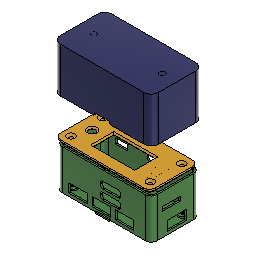
Raspi Zero 2W Case Zero4U V1.0 (Autodesk Fusion 360 design; units mm, degrees)
Autodesk Fusion 360 part; units mm, degrees
sketch "Skizze1" plane through (0, 0, 0) normal (0, 0, 1) x (1, 0, 0)
  line L0 (3, 0) -> (64, 0)
  line L1 (67, 3) -> (67, 30)
  line L2 (64, 33) -> (3, 33)
  line L3 (0, 30) -> (0, 3)
  arc A0 (3, 33) -> (0, 30) centre (3, 30) ccw
  arc A1 (67, 30) -> (64, 33) centre (64, 30) ccw
  arc A2 (64, 0) -> (67, 3) centre (64, 3) ccw
  arc A3 (0, 3) -> (3, 0) centre (3, 3) ccw
  line L4 (-1.2, 30) -> (-1.2, 3)
  arc A4 (-1.2, 3) -> (3, -1.2) centre (3, 3) ccw
  line L5 (3, -1.2) -> (64, -1.2)
  arc A5 (64, -1.2) -> (68.2, 3) centre (64, 3) ccw
  line L6 (68.2, 3) -> (68.2, 30)
  arc A6 (68.2, 30) -> (64, 34.2) centre (64, 30) ccw
  line L7 (64, 34.2) -> (3, 34.2)
  arc A7 (3, 34.2) -> (-1.2, 30) centre (3, 30) ccw
  point P0 (67, 0)
  point P1 (0, 33)
  dimension "d7" = 67
  dimension "d8" = 33
  dimension "d9" = 3
  dimension "d10" = 1.2
  constraint horizontal L0
  constraint vertical L1
  constraint horizontal L2
  constraint vertical L3
  constraint coincident P1 L2
  constraint coincident P1 L3
  constraint tangent L2 A0
  constraint tangent L3 A0
  constraint tangent L1 A1
  constraint tangent L2 A1
  constraint equal A0 A1
  constraint coincident P0 L0
  constraint coincident P0 L1
  constraint tangent L0 A2
  constraint tangent L1 A2
  constraint equal A0 A2
  constraint coincident origin L0
  constraint coincident origin L3
  constraint tangent L0 A3
  constraint tangent L3 A3
  constraint equal A0 A3
  measures "d7" distance of origin P0
  measures "d8" distance of origin P1
  measures "d9" radius of A0
extrude "Extrusion2" add sketch "Skizze1" against normal blind 1.2 contours L0 L1 L2 L3 A0 A1 A2 A3 | L4 A4 L5 A5 L6 A6 L7 A7 makes body 1
extrude "Extrusion3" add sketch "Skizze1" along normal blind 28 bodies 1
ref_plane "Arbeitsebene1" through (70.2, 0, 0) normal (1, 0, 0) x (0, 1, 0)
sketch "Skizze2" plane through (70.2, 0, 0) normal (1, 0, 0) x (0, 1, 0)
  line L0 (7, 18.5) -> (20, 18.5)
  line L1 (20, 18.5) -> (20, 15.5)
  line L2 (20, 15.5) -> (7, 15.5)
  line L3 (7, 15.5) -> (7, 18.5)
  line L4 (3, 0) -> (30, 0)
  line L5 (10.75, 8) -> (24.25, 8)
  line L6 (24.25, 8) -> (24.25, 1)
  line L7 (24.25, 1) -> (10.75, 1)
  line L8 (10.75, 1) -> (10.75, 8)
  line L9 (17.5, 35) -> (17.5, -5) construction
  point P0 (33, 0)
  dimension "d18" = 15.5
  dimension "d19" = 7
  dimension "d20" = 13.5
  dimension "d23" = 17.5
  dimension "d27" = 7
  dimension "d60" = 3
  dimension "d140" = 1
  constraint horizontal L0
  constraint vertical L1
  constraint horizontal L2
  constraint vertical L3
  constraint horizontal L5
  constraint vertical L6
  constraint horizontal L7
  constraint vertical L8
  constraint perpendicular L7 L9
  measures "d18" distance of L2.end L4
  measures "d19" horizontal distance of origin L2.end
  measures "d20" distance of L5.start L5.end
  measures "d23" distance of origin L9
  measures "d27" distance of L5.end L6.end
  measures "d60" distance of L0 L2
  measures "d140" distance of L4 L7
extrude "Extrusion4" cut sketch "Skizze2" against normal blind 3.2 bodies 1
ref_plane "Arbeitsebene2" through (-3.2, 0, 0) normal (1, 0, 0) x (0, 1, 0)
sketch "Skizze3" plane through (-3.2, 0, 0) normal (1, 0, 0) x (0, 1, 0)
  line L0 (16, 30) -> (16, -12) construction
  line L1 (23, 17) -> (25, 17)
  line L2 (25, 17) -> (25, 22)
  line L3 (25, 22) -> (23, 22)
  line L4 (23, 22) -> (23, 17)
  point P0 (33, 0)
  dimension "d166" = 17
  constraint horizontal L1
  constraint vertical L2
  constraint horizontal L3
  constraint vertical L4
  measures "d166" vertical distance of origin L1.end
extrude "Extrusion5" cut sketch "Skizze3" along normal blind 3.2 bodies 1
ref_plane "Arbeitsebene3" through (33.5, 36.2, 13.4) normal (0, 1, 0) x (1, 0, 0)
sketch "Skizze4" plane through (0, 36.2, 0) normal (0, 1, 0) x (1, 0, 0)
  line L0 (33.5, -32) -> (33.5, 14) construction
  line L1 (44, -21) -> (33, -21)
  line L2 (31, -19) -> (31, -18)
  line L3 (33, -16) -> (44, -16)
  line L4 (46, -18) -> (46, -19)
  line L5 (67, 0) -> (67, -28)
  line L6 (64, 0) -> (3, 0)
  line L7 (44, -9) -> (33, -9)
  line L8 (31, -11) -> (31, -12)
  line L9 (33, -14) -> (44, -14)
  line L10 (46, -12) -> (46, -11)
  arc A0 (44, -21) -> (46, -19) centre (44, -19) ccw
  arc A1 (31, -19) -> (33, -21) centre (33, -19) ccw
  arc A2 (33, -16) -> (31, -18) centre (33, -18) ccw
  arc A3 (46, -18) -> (44, -16) centre (44, -18) ccw
  arc A4 (46, -11) -> (44, -9) centre (44, -11) ccw
  arc A5 (33, -9) -> (31, -11) centre (33, -11) ccw
  arc A6 (31, -12) -> (33, -14) centre (33, -12) ccw
  arc A7 (44, -14) -> (46, -12) centre (44, -12) ccw
  line L11 (17, -19) -> (8, -19)
  line L12 (8, -19) -> (8, -15)
  line L13 (8, -15) -> (17, -15)
  line L14 (17, -15) -> (17, -19)
  line L15 (0, 0) -> (0, -28)
  point P0 (46, -21)
  point P1 (31, -21)
  point P2 (46, -16)
  point P3 (46, -9)
  point P4 (31, -9)
  dimension "d33" = 33.5
  dimension "d61" = 15
  dimension "d62" = 5
  dimension "d63" = 21
  dimension "d64" = 16
  dimension "d65" = 15
  dimension "d66" = 21
  dimension "d69" = 2
  dimension "d154" = 9
  dimension "d155" = 9
  dimension "d156" = 4
  dimension "d157" = 15
  dimension "d158" = 8
  constraint horizontal L1
  constraint vertical L2
  constraint horizontal L3
  constraint vertical L4
  constraint horizontal L7
  constraint vertical L8
  constraint horizontal L9
  constraint vertical L10
  constraint coincident P0 L1
  constraint coincident P0 L4
  constraint tangent L1 A0
  constraint tangent L4 A0
  constraint coincident P1 L1
  constraint coincident P1 L2
  constraint tangent L1 A1
  constraint tangent L2 A1
  constraint equal A0 A1
  constraint tangent L2 A2
  constraint tangent L3 A2
  constraint equal A0 A2
  constraint coincident P2 L3
  constraint coincident P2 L4
  constraint tangent L3 A3
  constraint tangent L4 A3
  constraint equal A0 A3
  constraint coincident P3 L7
  constraint coincident P3 L10
  constraint tangent L7 A4
  constraint tangent L10 A4
  constraint equal A0 A4
  constraint coincident P4 L7
  constraint coincident P4 L8
  constraint tangent L7 A5
  constraint tangent L8 A5
  constraint equal A0 A5
  constraint tangent L8 A6
  constraint tangent L9 A6
  constraint equal A0 A6
  constraint tangent L9 A7
  constraint tangent L10 A7
  constraint equal A0 A7
  constraint horizontal L11
  constraint vertical L12
  constraint horizontal L13
  constraint vertical L14
  measures "d33" distance of L15.start L0
  measures "d61" distance of P0 P1
  measures "d62" distance of P0 P2
  measures "d63" distance of L4 L5
  measures "d64" distance of L3 L6
  measures "d65" distance of P3 P4
  measures "d66" distance of L5 L10
  measures "d69" radius of A0
  measures "d154" distance of L6 L7.start
  measures "d155" distance of L11.start L11.end
  measures "d156" distance of L11.start L13.end
  measures "d157" distance of L6 L12.end
  measures "d158" distance of L11.end L15
extrude "Extrusion7" cut sketch "Skizze4" against normal blind 3.2 contours L1 L2 L3 L4 A0 A1 A2 A3 | L7 L8 L9 L10 A4 A5 A6 A7 bodies 1
sketch "Skizze5" plane through (0, 0, 0) normal (0, 0, 1) x (1, 0, 0)
  line L0 (1, 31.5) -> (66, 31.5)
  line L1 (66, 31.5) -> (66, 1.5)
  line L2 (66, 1.5) -> (1, 1.5)
  line L3 (1, 1.5) -> (1, 31.5)
  circle A0 centre (4.5, 28) radius 2.5
  circle A1 centre (62.5, 28) radius 2.5
  circle A2 centre (4.5, 5) radius 2.5
  circle A3 centre (62.5, 5) radius 2.5
  circle A4 centre (4.5, 28) radius 3.5
  circle A5 centre (62.5, 28) radius 3.5
  circle A6 centre (4.5, 5) radius 3.5
  circle A7 centre (62.5, 5) radius 3.5
  circle A8 centre (4.5, 28) radius 1.35
  circle A9 centre (62.5, 28) radius 1.35
  circle A10 centre (62.5, 5) radius 1.35
  circle A11 centre (4.5, 5) radius 1.35
  dimension "d40" = 30
  dimension "d41" = 65
  dimension "d42" = 5
  dimension "d43" = 3.5
  dimension "d44" = 3.5
  dimension "d45" = 5
  dimension "d46" = 3.5
  dimension "d47" = 3.5
  dimension "d48" = 5
  dimension "d49" = 3.5
  dimension "d50" = 3.5
  dimension "d51" = 5
  dimension "d52" = 3.5
  dimension "d53" = 3.5
  dimension "d54" = 7
  dimension "d55" = 7
  dimension "d56" = 7
  dimension "d57" = 7
  dimension "d114" = 2.7
  dimension "d115" = 2.7
  dimension "d116" = 2.7
  dimension "d117" = 2.7
  dimension "d162" = 1.5
  dimension "d165" = 1
  constraint horizontal L0
  constraint vertical L1
  constraint horizontal L2
  constraint vertical L3
  constraint concentric A0 A4
  constraint concentric A1 A5
  constraint concentric A2 A6
  constraint concentric A3 A7
  constraint concentric A4 A8
  constraint concentric A1 A9
  constraint concentric A7 A10
  constraint concentric A6 A11
  measures "d40" distance of L0.start L2.end
  measures "d41" distance of L1.end L2.end
  measures "d42" diameter of A0
  measures "d43" distance of L3 A0.centre
  measures "d44" distance of L0 A0.centre
  measures "d45" diameter of A1
  measures "d46" distance of L0 A1.centre
  measures "d47" distance of L1 A1.centre
  measures "d48" diameter of A2
  measures "d49" distance of L3 A2.centre
  measures "d50" distance of L2 A2.centre
  measures "d51" diameter of A3
  measures "d52" distance of L2 A3.centre
  measures "d53" distance of L1 A3.centre
  measures "d54" diameter of A4
  measures "d55" diameter of A5
  measures "d56" diameter of A6
  measures "d57" diameter of A7
  measures "d114" diameter of A8
  measures "d115" diameter of A11
  measures "d116" diameter of A10
  measures "d117" diameter of A9
  measures "d162" vertical distance of origin L2.end
  measures "d165" horizontal distance of origin L2.end
extrude "Extrusion18" add sketch "Skizze5" along normal blind 1 contours A4 | A5 | A6 | A7 | A0 | A1 | A2 | A3 bodies 1
extrude "Extrusion19" cut sketch "Skizze5" against normal blind 1.2 contours A8 | A9 | A10 | A11 bodies 1
chamfer "Fase4" distance 1.4 angle 45 2 edges at (61.2414, 4.5118, -1.2) (3.2414, 27.5118, -1.2) on bodies 1
chamfer "Fase4" distance 1.4 angle 45 2 edges at (61.2414, 27.5118, -1.2) (3.2414, 4.5118, -1.2) on bodies 1
extrude "Extrusion9" cut sketch "Skizze4" against normal blind 42 contours L1 L2 L3 L4 A0 A1 A2 A3 | L7 L8 L9 L10 A4 A5 A6 A7 bodies 1
ref_plane "Arbeitsebene4" through (33.5, 16.5, 30) normal (0, 0, 1) x (1, 0, 0)
sketch "Skizze6" plane through (0, 0, 30) normal (0, 0, 1) x (1, 0, 0)
  arc A0 (3, 34.2) -> (-1.2, 30) centre (3, 30) ccw
  line L0 (64, 34.2) -> (3, 34.2)
  line L1 (68.2, 3) -> (68.2, 30)
  arc A1 (68.2, 30) -> (64, 34.2) centre (64, 30) ccw
  arc A2 (64, -1.2) -> (68.2, 3) centre (64, 3) ccw
  line L2 (3, -1.2) -> (64, -1.2)
  arc A3 (-1.2, 3) -> (3, -1.2) centre (3, 3) ccw
  line L3 (-1.2, 30) -> (-1.2, 3)
  line L4 (0, 30) -> (0, 3)
  arc A4 (3, 33) -> (0, 30) centre (3, 30) ccw
  line L5 (64, 33) -> (3, 33)
  arc A5 (67, 30) -> (64, 33) centre (64, 30) ccw
  line L6 (67, 3) -> (67, 30)
  arc A6 (64, 0) -> (67, 3) centre (64, 3) ccw
  line L7 (3, 0) -> (64, 0)
  arc A7 (0, 3) -> (3, 0) centre (3, 3) ccw
  line L8 (1.25, 30) -> (1.25, 3)
  arc A8 (1.25, 3) -> (3, 1.25) centre (3, 3) ccw
  line L9 (3, 1.25) -> (64, 1.25)
  arc A9 (64, 1.25) -> (65.75, 3) centre (64, 3) ccw
  line L10 (65.75, 3) -> (65.75, 30)
  arc A10 (65.75, 30) -> (64, 31.75) centre (64, 30) ccw
  line L11 (64, 31.75) -> (3, 31.75)
  arc A11 (3, 31.75) -> (1.25, 30) centre (3, 30) ccw
  line L12 (0.05, 30) -> (0.05, 3)
  arc A12 (0.05, 3) -> (3, 0.05) centre (3, 3) ccw
  line L13 (3, 0.05) -> (64, 0.05)
  arc A13 (64, 0.05) -> (66.95, 3) centre (64, 3) ccw
  line L14 (66.95, 3) -> (66.95, 30)
  arc A14 (66.95, 30) -> (64, 32.95) centre (64, 30) ccw
  line L15 (64, 32.95) -> (3, 32.95)
  arc A15 (3, 32.95) -> (0.05, 30) centre (3, 30) ccw
  line L16 (18.55, 25.5) -> (48.65, 25.5)
  line L17 (48.65, 25.5) -> (48.65, 10.5)
  line L18 (48.65, 10.5) -> (18.55, 10.5)
  line L19 (18.55, 10.5) -> (18.55, 25.5)
  line L20 (1, 31.5) -> (66, 31.5)
  line L21 (-5, 16.5) -> (70.5561, 16.5) construction
  circle A16 centre (58.5, 16.5) radius 2.5
  line L22 (6, 19.7) -> (12, 19.7)
  line L23 (12, 19.7) -> (12, 15.7)
  line L24 (12, 15.7) -> (6, 15.7)
  line L25 (6, 15.7) -> (6, 19.7)
  line L26 (6, 26) -> (12, 26)
  line L27 (12, 22) -> (6, 22)
  line L28 (12, 26) -> (12, 22)
  line L29 (6, 22) -> (6, 26)
  line L30 (12, 13.4) -> (12, 9.4)
  line L31 (12, 9.4) -> (6, 9.4)
  line L32 (6, 13.4) -> (12, 13.4)
  line L33 (6, 9.4) -> (6, 13.4)
  circle A17 centre (62.5, 28) radius 1.35
  circle A18 centre (62.5, 5) radius 1.35
  circle A19 centre (4.5, 28) radius 1.35
  circle A20 centre (4.5, 5) radius 1.35
  circle A21 centre (62.5, 28) radius 2.5
  circle A22 centre (62.5, 5) radius 2.5
  circle A23 centre (4.5, 5) radius 2.5
  circle A24 centre (4.5, 28) radius 2.5
  point P0 (62.5, 28)
  point P1 (62.5, 5)
  point P2 (4.5, 5)
  point P3 (4.5, 28)
  dimension "d80" = 18.5
  dimension "d81" = 6
  dimension "d83" = 5
  dimension "d84" = 8.5
  dimension "d90" = 16.5
  dimension "d92" = 12
  dimension "d95" = 12
  dimension "d96" = 12
  dimension "d97" = 7
  dimension "d98" = 2.3
  dimension "d99" = 4
  dimension "d100" = 4
  dimension "d101" = 2.3
  dimension "d102" = 4
  dimension "d103" = 15
  dimension "d104" = 2.7
  dimension "d105" = 2.7
  dimension "d106" = 2.7
  dimension "d107" = 2.7
  constraint horizontal L16
  constraint vertical L17
  constraint horizontal L18
  constraint vertical L19
  constraint perpendicular L1 L21
  constraint coincident L21 A16.centre
  constraint horizontal L22
  constraint vertical L23
  constraint horizontal L24
  constraint vertical L25
  constraint horizontal L26
  constraint vertical L28
  constraint horizontal L27
  constraint vertical L29
  constraint horizontal L32
  constraint vertical L30
  constraint horizontal L31
  constraint vertical L33
  constraint coincident P0 A17.centre
  constraint coincident P1 A18.centre
  constraint coincident P3 A19.centre
  constraint coincident P2 A20.centre
  measures "d80" distance of L12 L19
  measures "d81" distance of L16 L20
  measures "d83" diameter of A16
  measures "d84" distance of L6 A16.centre
  measures "d90" distance of L5 A16.centre
  measures "d92" distance of L4 L23
  measures "d95" distance of L4 L30
  measures "d96" distance of L4 L28
  measures "d97" distance of L5 L26
  measures "d98" distance of L22 L27
  measures "d99" distance of L26 L27
  measures "d100" distance of L22 L24
  measures "d101" distance of L24 L32
  measures "d102" distance of L31 L32
  measures "d103" distance of L16 L18
  measures "d104" diameter of A17
  measures "d105" diameter of A18
  measures "d106" diameter of A19
  measures "d107" diameter of A20
extrude "Extrusion11" add sketch "Skizze6" along normal blind 1.2 separate body contours A0 L0 L1 A1 A2 L2 A3 L3 | L4 A4 L5 A5 L6 A6 L7 A7 | L8 A8 L9 A9 L10 A10 A11 L20 | A10 L11 A11 L20 | L12 A12 L13 A13 L14 A14 L15 A15 | L16 L17 L18 L19 | A16 | L22 L23 L24 L25 | L26 L27 L28 L29 | A24 | L30 L31 L32 L33 | A17 | A18 | A19 | A20 | A21 | A22 | A23 makes body 2
extrude "Extrusion12" add sketch "Skizze6" against normal blind 1.5 contours L12 A12 L13 A13 L14 A14 L15 A15 bodies 2
sketch "Skizze7" plane through (0, 0, 31.2) normal (0, 0, 1) x (-1, 0, 0)
  line L0 (1.2, -30) -> (1.2, -3)
  arc A0 (1.2, -3) -> (-3, 1.2) centre (-3, -3) ccw
  line L1 (-3, 1.2) -> (-64, 1.2)
  arc A1 (-64, 1.2) -> (-68.2, -3) centre (-64, -3) ccw
  line L2 (-68.2, -3) -> (-68.2, -30)
  arc A2 (-68.2, -30) -> (-64, -34.2) centre (-64, -30) ccw
  line L3 (-64, -34.2) -> (-3, -34.2)
  arc A3 (-3, -34.2) -> (1.2, -30) centre (-3, -30) ccw
extrude "Extrusion13" cut sketch "Skizze6" along normal blind 1.2 contours L16 L17 L18 L19 bodies 2
extrude "Extrusion14" cut sketch "Skizze6" along normal blind 1.2 contours A16 bodies 2
chamfer "Fase1" distance 1 angle 45 4 edges at (33.6, 25.5, 31.2) (48.65, 18, 31.2) (33.6, 10.5, 31.2) (18.55, 18, 31.2) on bodies 2
extrude "Extrusion15" cut sketch "Skizze6" along normal blind 0.6 contours L22 L23 L24 L25 | L26 L27 L28 L29 | L30 L31 L32 L33 bodies 2
extrude "Extrusion16" cut sketch "Skizze6" along normal blind 1.2 contours A17 | A18 | A19 | A20 bodies 2
extrude "Extrusion17" add sketch "Skizze6" against normal blind 2 contours A24 | A21 | A22 | A23 bodies 2
chamfer "Fase2" distance 1 angle 45 1 edges at (56.1692, 17.404, 31.2) on bodies 2
chamfer "Fase3" distance 1.4 angle 45 4 edges at (61.2414, 28.4882, 31.2) (61.2414, 5.4882, 31.2) (3.2414, 5.4882, 31.2) (3.2414, 28.4882, 31.2) on bodies 2
ref_plane "Arbeitsebene5" through (33.5, 16.5, 32) normal (0, 0, 1) x (1, 0, 0)
sketch "Skizze8" plane through (0, 0, 32) normal (0, 0, 1) x (1, 0, 0)
  line L0 (64, 34.2) -> (3, 34.2)
  arc A0 (3, 34.2) -> (-1.2, 30) centre (3, 30) ccw
  line L1 (-1.2, 30) -> (-1.2, 3)
  arc A1 (-1.2, 3) -> (3, -1.2) centre (3, 3) ccw
  line L2 (3, -1.2) -> (64, -1.2)
  arc A2 (64, -1.2) -> (68.2, 3) centre (64, 3) ccw
  line L3 (68.2, 3) -> (68.2, 30)
  arc A3 (68.2, 30) -> (64, 34.2) centre (64, 30) ccw
  line L4 (-2.45, 30) -> (-2.45, 3)
  arc A4 (-2.45, 3) -> (3, -2.45) centre (3, 3) ccw
  line L5 (3, -2.45) -> (64, -2.45)
  arc A5 (64, -2.45) -> (69.45, 3) centre (64, 3) ccw
  line L6 (69.45, 3) -> (69.45, 30)
  arc A6 (69.45, 30) -> (64, 35.45) centre (64, 30) ccw
  line L7 (64, 35.45) -> (3, 35.45)
  arc A7 (3, 35.45) -> (-2.45, 30) centre (3, 30) ccw
  line L8 (-1.3, 30) -> (-1.3, 3)
  arc A8 (-1.3, 3) -> (3, -1.3) centre (3, 3) ccw
  line L9 (3, -1.3) -> (64, -1.3)
  arc A9 (64, -1.3) -> (68.3, 3) centre (64, 3) ccw
  line L10 (68.3, 3) -> (68.3, 30)
  arc A10 (68.3, 30) -> (64, 34.3) centre (64, 30) ccw
  line L11 (64, 34.3) -> (3, 34.3)
  arc A11 (3, 34.3) -> (-1.3, 30) centre (3, 30) ccw
  circle A12 centre (58.5071, 16.5) radius 2
  line L12 (33.5, 50) -> (33.5, -6)
  line L13 (33.5, 50) -> (33.5, -6)
  circle A13 centre (8.4929, 16.5) radius 2
  dimension "d126" = 1.25
  dimension "d127" = 0.1
  dimension "d132" = 4
  dimension "d170" = 18.95
  dimension "d171" = 37.9
  dimension "d205" = 71.9
  dimension "d206" = 35.95
  constraint perpendicular L5 L12
  constraint symmetric A12 L12 A13
  constraint symmetric L13.start L12 L12.start
  constraint symmetric L13.end L12 L12.end
  measures "d132" diameter of A12
  measures "d170" distance of L7 A12.centre
  measures "d171" distance of L5 L7
  measures "d205" distance of L4 L6
  measures "d206" distance of L4 L12
extrude "Extrusion20" add sketch "Skizze8" against normal blind 30.4 separate body contours L5 A5 L6 A6 L7 L9 A9 L10 A10 L11 L12 L13 | L4 A4 L5 L7 A7 L8 A8 L9 L11 A11 L12 L13 makes body 3
extrude "Extrusion21" add sketch "Skizze8" along normal blind 2.4 contours L0 L2 A2 L3 A3 L12 L13 | L0 L2 A2 L3 A3 L9 A9 L10 A10 L11 L12 L13 | L0 A0 L1 A1 L2 L12 L13 | L0 A0 L1 A1 L2 L8 A8 L9 L11 A11 L12 L13 | L5 A5 L6 A6 L7 L9 A9 L10 A10 L11 L12 L13 | L4 A4 L5 L7 A7 L8 A8 L9 L11 A11 L12 L13 | A12 | A13 bodies 3
extrude "Extrusion22" cut sketch "Skizze8" along normal blind 2 contours A12 | A13 bodies 3
copy_body "Körper->Berechn1" bodies 1 removing the originals makes body 4 in component "LBB_RaspiZero2W_bottom_zero4u"
copy_body "Körper->Berechn2" bodies 2 removing the originals makes body 5 in component "LBB_RaspiZero2W_top_zero4u"
copy_body "Körper->Berechn3" bodies 3 removing the originals makes body 6 in component "LBB_RaspiZero2W_cover_zero4u"
ref_plane "Arbeitsebene6" through (33.5, -3.2, 13.4) normal (0, -1, 0) x (-1, 0, 0)
sketch "Skizze10" plane through (0, -3.2, 0) normal (0, -1, 0) x (-1, 0, 0)
  line L0 (-8, -1) -> (-21.5, -1)
  line L1 (-21.5, -1) -> (-21.5, -7.5)
  line L2 (-21.5, -7.5) -> (-8, -7.5)
  line L3 (-8, -7.5) -> (-8, -1)
  line L4 (-3, 0) -> (-64, 0)
  line L5 (0, 0) -> (0, -28)
  line L6 (-25, -1) -> (-38.5, -1)
  line L7 (-38.5, -1) -> (-38.5, -7.5)
  line L8 (-38.5, -7.5) -> (-25, -7.5)
  line L9 (-25, -7.5) -> (-25, -1)
  line L10 (-42, -1) -> (-55.5, -1)
  line L11 (-55.5, -1) -> (-55.5, -7.5)
  line L12 (-55.5, -7.5) -> (-42, -7.5)
  line L13 (-42, -7.5) -> (-42, -1)
  dimension "d142" = 13.5
  dimension "d143" = 6.5
  dimension "d144" = 1
  dimension "d145" = 8
  dimension "d146" = 13.5
  dimension "d147" = 6.5
  dimension "d148" = 3.5
  dimension "d149" = 6.5
  dimension "d150" = 13.5
  dimension "d151" = 3.5
  constraint horizontal L0
  constraint vertical L1
  constraint horizontal L2
  constraint vertical L3
  constraint horizontal L6
  constraint vertical L7
  constraint horizontal L8
  constraint vertical L9
  constraint horizontal L10
  constraint vertical L11
  constraint horizontal L12
  constraint vertical L13
  measures "d142" distance of L0.start L0.end
  measures "d143" distance of L0.end L1.end
  measures "d144" distance of L0.end L4
  measures "d145" distance of L2.end L5
  measures "d146" distance of L6.start L6.end
  measures "d147" distance of L6.start L8.end
  measures "d148" distance of L1.end L8.end
  measures "d149" distance of L10.start L12.end
  measures "d150" distance of L10.start L10.end
  measures "d151" distance of L7.end L12.end
extrude "Extrusion1" cut sketch "Skizze10" against normal blind 3.2 bodies 4 in component "LBB_RaspiZero2W_bottom_zero4u"
extrude "Extrusion2'" cut sketch "Skizze4" against normal blind 3.2 contours L11 L12 L13 L14 bodies 4 in component "LBB_RaspiZero2W_bottom_zero4u"
ref_plane "Arbeitsebene7" through (33.5, 36.2, 13.4) normal (0, 1, 0) x (1, 0, 0)
ref_plane "Arbeitsebene8" through (33.5, -2.45, 13.4) normal (0, 1, 0) x (1, 0, 0)
ref_plane "Arbeitsebene9" through (33.5, 37.45, 55) normal (0, 1, 0) x (1, 0, 0)
sketch "Skizze11" plane through (0, 37.45, 0) normal (0, 1, 0) x (1, 0, 0)
  line L0 (69.45, -38.6) -> (69.45, -71.4)
  line L1 (33.5, -88) -> (33.5, -36) construction
  line L2 (3, -38.6) -> (64, -38.6) construction
  circle A0 centre (33.5, -38.6) radius 5
  point P0 (-2.45, -71.4)
  dimension "d176" = 71.9
  dimension "d177" = 35.95
  dimension "d179" = 10
  constraint vertical L1
  constraint midpoint L2 A0.centre
  measures "d176" distance of L0.end P0
  measures "d177" distance of P0 L1
  measures "d179" diameter of A0
extrude "Extrusion1'" cut sketch "Skizze11" against normal blind 3.2 sketch seen with x (1, 0, 0) y (0, 1, 0) z (0, 0, 1) at (0, 0, -37) bodies 6 in component "LBB_RaspiZero2W_cover_zero4u"
fillet "Abrundung1" radius 1 2 edges at (38.5, 34.875, 1.6) (28.5, 34.875, 1.6) on bodies 6 in component "LBB_RaspiZero2W_cover_zero4u"
ref_plane "Arbeitsebene10" through (33.5, -4.45, 55) normal (0, -1, 0) x (-1, 0, 0)
sketch "Skizze12" plane through (0, -4.45, 0) normal (0, -1, 0) x (-1, 0, 0)
  line L0 (-33.5, -84) -> (-33.5, -35) construction
  line L1 (-64, -38.6) -> (-3, -38.6) construction
  line L2 (2.45, -38.6) -> (2.45, -71.4) construction
  line L3 (-28, -40.6) -> (-39, -40.6)
  line L4 (-39, -40.6) -> (-39, -38.6)
  line L5 (-39, -38.6) -> (-28, -38.6)
  line L6 (-28, -38.6) -> (-28, -40.6)
  point P0 (-69.45, -71.4)
  dimension "d186" = 71.9
  dimension "d187" = 35.95
  dimension "d188" = 2
  dimension "d189" = 11
  dimension "d191" = 2
  constraint vertical L0
  constraint horizontal L3
  constraint vertical L4
  constraint horizontal L5
  constraint vertical L6
  constraint symmetric L0 L4 L6
  measures "d186" distance of L2.end P0
  measures "d187" distance of L0 L2.end
  measures "d188" distance of L3.start L5.end
  measures "d189" distance of L3.start L3.end
  measures "d191" distance of L1 L3
extrude "Extrusion2''" cut sketch "Skizze12" against normal blind 3.2 sketch seen with x (1, 0, 0) y (0, 1, 0) z (0, 0, 1) at (0, 0, -37) bodies 6 in component "LBB_RaspiZero2W_cover_zero4u"
fillet "Abrundung2" radius 1 2 edges at (28, -1.875, 1.6) (39, -1.875, 1.6) on bodies 6 in component "LBB_RaspiZero2W_cover_zero4u"
ref_plane "Arbeitsebene11" through (33.5, -1.2, 13.4) normal (0, -1, 0) x (-1, 0, 0)
sketch "Skizze13" plane through (0, -1.2, 0) normal (0, -1, 0) x (-1, 0, 0)
  line L0 (-33.5, -35) -> (-33.5, 13) construction
  line L1 (1.2, 1.2) -> (1.2, -28) construction
  line L2 (-64, 1.2) -> (-3, 1.2)
  line L3 (-28.5, 1.2) -> (-38.5, 1.2)
  line L4 (-38.5, 1.2) -> (-38.5, 0.2)
  line L5 (-38.5, 0.2) -> (-28.5, 0.2)
  line L6 (-28.5, 0.2) -> (-28.5, 1.2)
  point P0 (1.2, 1.2)
  point P1 (-68.2, -28)
  dimension "d198" = 34.7
  dimension "d200" = 69.4
  dimension "d201" = 1
  dimension "d202" = 10
  constraint vertical L0
  constraint horizontal L3
  constraint vertical L4
  constraint horizontal L5
  constraint vertical L6
  constraint coincident L2 L3.start
  constraint symmetric L0 L4 L6
  measures "d198" distance of L0 P0
  measures "d200" distance of L1.end P1
  measures "d201" distance of L3.start L5.end
  measures "d202" distance of L3.start L3.end
extrude "Extrusion3'" add sketch "Skizze13" along normal blind 1 bodies 4 in component "LBB_RaspiZero2W_bottom_zero4u"
component "LBB_RaspiZero2W_bottom_zero4u" placed x (1, 0, 0) y (0, 1, 0) z (0, 0, 1) at (0, 0, 0)
component "LBB_RaspiZero2W_top_zero4u" placed x (1, 0, 0) y (0, 1, 0) z (0, 0, 1) at (0, 0, 1)
component "LBB_RaspiZero2W_cover_zero4u" placed x (1, 0, 0) y (0, 1, 0) z (0, 0, 1) at (0, 0, 37)
equation "breite = 33 mm"
equation "länge = 67 mm"
equation "höhe = 28 mm"
equation "wanddicke = 1.2 mm"
equation "radius = 3 mm"
equation "d7 = länge"
equation "d8 = breite"
equation "d9 = radius"
equation "d10 = wanddicke"
equation "d13 = -wanddicke"
equation "d15 = höhe"
equation "d17 = länge + wanddicke + abstand_ebene"
equation "d23 = breite / 2 + 1 mm"
equation "d24 = -( wanddicke + abstand_ebene )"
equation "abstand_ebene = 2 mm"
equation "d28 = -( wanddicke + abstand_ebene )"
equation "d30 = abstand_ebene + wanddicke"
equation "d32 = ( abstand_ebene )"
equation "d33 = länge / 2"
equation "d37 = -( abstand_ebene + wanddicke )"
equation "d40 = board_breite"
equation "d41 = board_laenge"
equation "d45 = d42"
equation "d46 = d44"
equation "d47 = d43"
equation "d48 = d42"
equation "d49 = d43"
equation "d50 = d44"
equation "d51 = d42"
equation "d52 = d44"
equation "d53 = d43"
equation "d55 = d54"
equation "d56 = d54"
equation "d57 = d54"
equation "d66 = d63"
equation "d72 = abstand_ebene"
equation "gap = 0.05 mm"
equation "d74 = -( wanddicke + gap )"
equation "d75 = -gap"
equation "d76 = wanddicke"
equation "d85 = wanddicke"
equation "d87 = wanddicke"
equation "d90 = breite / 2"
equation "d93 = wanddicke - 0.6 mm"
equation "d95 = d92"
equation "d96 = d92"
equation "d105 = d104"
equation "d106 = d104"
equation "d107 = d104"
equation "d108 = wanddicke"
equation "d113 = schrauben_fase"
equation "d115 = d114"
equation "d116 = d114"
equation "d117 = d114"
equation "d120 = -wanddicke"
equation "d122 = schrauben_fase"
equation "d123 = schrauben_fase"
equation "schrauben_fase = 1.4 mm"
equation "d126 = wanddicke + gap"
equation "d127 = 2 * gap"
equation "d128 = -( höhe + wanddicke * 2 )"
equation "d130 = wanddicke * 2"
equation "d143 = d147"
equation "d146 = d142"
equation "d149 = d147"
equation "d150 = d146"
equation "d151 = d148"
equation "d152 = -( 2 mm + wanddicke )"
equation "d159 = -( 2 mm + wanddicke )"
equation "d162 = ( breite - board_breite ) / 2"
equation "board_breite = 30 mm"
equation "board_laenge = 65 mm"
equation "d165 = ( länge - board_laenge ) / 2"
equation "d170 = d171 / 2"
equation "d172 = abstand_ebene"
equation "d174 = abstand_ebene"
equation "d177 = d176 / 2"
equation "d180 = -( abstand_ebene + wanddicke )"
equation "d184 = abstand_ebene"
equation "d187 = d186 / 2"
equation "d188 = wanddicke + 0.8 mm"
equation "d191 = wanddicke + 0.8 mm"
equation "d192 = -( abstand_ebene + wanddicke )"
equation "d198 = d200 / 2"
equation "d206 = d205 / 2"
named bodies: "RaspiZero2W_bottom", "RaspiZero2W_top", "RaspiZero2W_cover", "RaspiZero2W_bottom_zero4u", "RaspiZero2W_top_zero4u", "RaspiZero2W_cover_zero4u"
